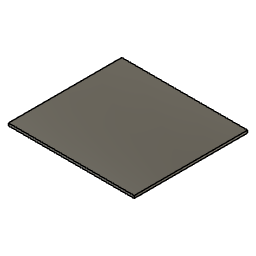
base_plate v1 (Autodesk Fusion 360 design; units mm, degrees)
Autodesk Fusion 360 part; units mm, degrees
sketch "Sketch1" plane through (0, 0, 0) normal (0, 0, 1) x (1, 0, 0)
  line L0 (0, 0) -> (302.2, 0)
  line L1 (302.2, 0) -> (302.2, 272.2)
  line L2 (302.2, 272.2) -> (0, 272.2)
  line L3 (0, 272.2) -> (0, 0)
  dimension "d1" = 302.2
  dimension "d2" = 272.2
  constraint horizontal L0
  constraint vertical L1
  constraint horizontal L2
  constraint vertical L3
  constraint coincident L0.start L3.end
  measures "d1" distance of L0.start L0.end
  measures "d2" distance of L0 L2
extrude "Extrude1" add sketch "Sketch1" against normal blind 6
